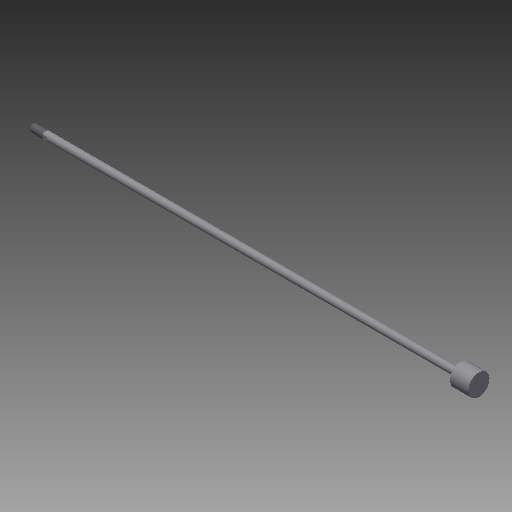
# Autodesk Inventor part: SR-1222-DP0000_rod
Saved by Autodesk Inventor 2019 (Build 230136000, 136)
## iProperties
Category: PARTsolutions
Company: BIMBA
Created: 2019-01-13
Part Number: SR-1222-DP0000_rod
Material: Generic
Catalog Web Link: www.cadenas.de
Description: Standard Air Cylinder_rod-Original Line - Standard Air Cylinders
Vendor: BIMBA
Document SubType Name: Modeling
Designer: psadmin
Manufacturer: BIMBA
Mass: 83.0612 g
Surface Area: 264.5 cm^2
Volume: 83.0612 cm^3
Density: 1 g/cm^3
Appearance: PSOLRGB-181-181-181
PSOL_IDENT_0: {$CADENAS_DATA\23d-libs\bimba\bimba\bimba_imperial\bimba_full_line\original_line_cylinders\standard_
PSOL_IDENT_1: air_cylinders\rod.prj},329 {VTYP=3D},{NB=SR-1222-DP0000_rod},{LINA=SR-1222-DP0000_rod},{NN=Standard
PSOL_IDENT_2: Air Cylinder_rod},{DATE=21.03.2018 14:31:21},{GEOMDATE=09.11.2017 13:09:15},{VERSION=},{LINEID=70},{
PSOL_IDENT_3: WBVAR=STROKE,ACTING,MNT,DER,NR,BM,CO,M,EE,EEL,K,Q,Y,F,G,T,B,H,SER,SR,NT,W,E,HL,ST,STP,PRC,PB,COLOR1,
PSOL_IDENT_4: FCD,RCD,BCD},{WBNUMERIC=STROKE,EEL,COLOR1,FCD,RCD,BCD}  {NB=SR-1222-DP0000_rod},{LINA=SR-1222-DP0000
PSOL_IDENT_5: _rod},{KT=DUMMY},{PN=SR-1222-DP000},{DASH=-},{BORE=1.25000000},{BOREPN=12},{STROKE=22.000},{STROKEAL
PSOL_IDENT_6: G=[0.001:50/0.001]},{STROKE1=22.000},{ACTING=D},{ACTINGALG= '' , 'Single Acting' , 'R' , 'Reverse Si
PSOL_IDENT_7: ngle Acting' , 'D' , 'Double Acting' },{ACTINGPN=D},{MNT=P},{MNTALG= '' , 'Front Nose Mounting' , 'P'
PSOL_IDENT_8: , 'Rear Pivot Mounting' , 'X' , 'Double End Mounting' },{TYPE=SR-},{MNTPN=P},{DER=},{DERALG= '' , '
PSOL_IDENT_9: N/A' },{NR=},{NRALG= '' , 'N/A' },{NRPN=},{BM=},{BMALG= '' , 'N/A' },{BMPN=},{CO=},{COALG= '' , 'N/A'
PSOL_IDENT_10: },{M=},{MALG= '', 'Without Magnet', 'M', 'With Magnet' },{EE=},{EEL=0},{EEMAX=28},{EEALG= '', 'With
PSOL_IDENT_11: out Extra Extension', 'EE', 'With Extra Extension' },{EELALG=0},{EEPN=},{EEPN1=0.000},{K=},{KALG= ''
PSOL_IDENT_12: , 'Standard' , 'K' , 'Ports Rotated 90deg' },{KPN=},{Q=},{QALG= '' , 'Without Side Ported Rear Head'
PSOL_IDENT_13: , 'Q' , 'With Side Ported Rear Head' },{QPN=},{Y=},{YALG= '' , 'Without Pivot Bushing' , 'Y' , 'Wit
PSOL_IDENT_14: h Pivot Bushing' },{YPN=},{F=},{FALG= '', 'Standard', 'F', 'Molycoated Body' },{FPN=},{G=},{GPN=},{T=
PSOL_IDENT_15: },{TALG= '' , 'Standard' , 'N' , 'Low Temperature' , 'V' , 'High Temperature' },{NPN=},{VPN=},{B=},{
PSOL_IDENT_16: BALG= '' , 'With Bumper' },{BPN=},{H=},{HALG= '', 'N/A' },{HPN=},{SER=},{SERALG= '' , 'Without Sprin
PSOL_IDENT_17: g Extend/Return' , 'JS' , 'With Spring Return' , 'JR' , 'With Spring Extend' },{SR=SR},{SRALG= 'C' ,
PSOL_IDENT_18: 'Carbon Steel Rod' , 'SR' , '303 Stainless Steel Rod' , '' , '303 Stainless Steel Rod1' },{SRPN=SR}
PSOL_IDENT_19: ,{SRCON=1},{NT=},{NTPN=},{W=},{WALG= '' , 'Without Wiper' , 'W' , 'With Wiper' },{WPN=},{E=},{EALG= ''
PSOL_IDENT_20: , 'Without Special Lube and Seals' , 'E' , 'With Special Lube and Seals' },{EPN=},{HL=},{HLALG= ''
PSOL_IDENT_21: , 'Wihout Low Pressure Hydraulic' , 'HL' , 'With Low Pressure Hydraulic' },{ST=},{STALG= '' , 'Witho
PSOL_IDENT_22: ut Switch Track' , 'T' , 'With Switch Track' },{STP=},{STPALG= '' , 'N/A' },{STPN=},{PRC=},{PRCALG= ''
PSOL_IDENT_23: , 'Without Piston Rod Clevis' , 'D-166-1' , 'With Piston Rod Clevis' },{PRCPN=},{PB=},{PBALG= '' , '
PSOL_IDENT_24: Without Pivot Bracket' , 'D-167' , 'With Pivot Bracket' },{PBPN=},{TLEN=23.4865},{TEXT=1.566667},{SP
PSOL_IDENT_25: ACE=0.895238},{FRAC=509.7200},{RGCON=},{RGDACCON=R},{RHCON=P},{RHCONON=1},{RHACCON=},{FNUTCON=1},{RN
PSOL_IDENT_26: UTCON=1},{FNUTPN=D-3556},{RNUTPN=D-3556},{FNUTTRANS=0.0000},{RNUTTRANS=0.0000},{VHOLECON=0},{A1=2.00
PSOL_IDENT_27: 00},{A1N=1.5620},{A1P=2.0000},{A1B=0.0000},{A4=0.2525},{A4N=0.6280},{A4P=0.2525},{A5=0.0400},{A1H=1.
PSOL_IDENT_28: 812},{A1NH=0.6880},{A1PH=1.8120},{A1BH=0.0000},{A1SH=1.1250},{A2H=0.2500},{A2NH=0.2500},{LENGTH=4.72
PSOL_IDENT_29: 00},{LENGTH1=4.7200},{LENGTH2=5.0900},{MUL=22.0000},{MUL11=22.0000},{MUL22=61.8200},{MUL33=39.8200},
PSOL_IDENT_30: {MUL2=22.0000},{MUL211=22.0000},{MUL222=2.8100},{MUL233=1.8100},{SSS=44.0000},{RGLEN=1.7875},{RHLEN=
PSOL_IDENT_31: 1.1960},{SSS1=23.0000},{A13=1.4060},{THDLEN1=0.7500},{THD1=0.4375},{TAB=UNF},{THDLEN=0.7500},{THD=0.
PSOL_IDENT_32: 4375},{OD=1.2615},{RODL=26.0640},{PL=1.0640},{RODDIA=0.4370},{HEX=0.4370},{RODTRANS=0.0000},{G1=0.37
PSOL_IDENT_33: 50},{ON=0},{G5=1.0000},{DERLEN=24.7500},{THOLE=0.2500},{WF=0.3800},{BADD=0.0000},{MADD=0.0000},{NVAD
PSOL_IDENT_34: D=0.000},{JRADD=0.00000},{COLOR=0.71,0.71,0.71,0.00},{GROOVE=1},{HOL=1},{D7=0.2525},{H1=1.3265},{D1=
PSOL_IDENT_35: 1.3265},{D1RH=1.3265},{D1P=0.0000},{D1B=1.3265},{D1N=1.3265},{D1NRH=1.3265},{D1BRH=0.0000},{D1PRH=1.
PSOL_IDENT_36: 3265},{BOZO=0},{HADD=0.000},{COLOR1=0},{DEFL=0.0000},{HEXL=0.0000},{SSADD=0.0000},{WFL=0.2500},{MOVE=
PSOL_IDENT_37: 0.2500},{PRCL2=0.75000},{PRCB=0.25000},{PRCTRANS=0.25000},{FCD=0},{RCD=0},{BCD=0}
NN: Standard Air Cylinder_rod
NT: Standard
NB: SR-1222-DP0000_rod
NBSYN: $PN.$COLOR1._rod
LINA: SR-1222-DP0000_rod
PN: SR-1222-DP000
BORE: 1.25
BOREPN: 12
STROKE: 22
ACTING: Double Acting
MNT: Rear Pivot Mounting
DER: N/A
NR: N/A
BM: N/A
CO: N/A
M: Without Magnet
EE: Without Extra Extension
EEL: 0
K: Standard
Q: Without Side Ported Rear Head
Y: Without Pivot Bushing
F: Standard
G: Without Magnalube Lubrication
T: Standard
B: With Bumper
H: N/A
SER: Without Spring Extend/Return
SR: 303 Stainless Steel Rod
W: Without Wiper
E: Without Special Lube and Seals
HL: Wihout Low Pressure Hydraulic
ST: Without Switch Track
STP: N/A
PRC: Without Piston Rod Clevis
PB: Without Pivot Bracket
A1N: 1.562
A1P: 2
A1B: 0
A4N: 0.628
A4P: 0.2525
A5: 0.04
A1NH: 0.688
A1PH: 1.812
A1BH: 0
A1SH: 1.125
A2NH: 0.25
A13: 1.406
THDLEN1: 0.75
THD1: 0.4375
TAB: UNF
OD: 1.2615
RODDIA: 0.437
HEX: 0.437
G1: 0.375
G5: 1
THOLE: 0.25
WF: 0.38
GROOVE: 1
D7: 0.2525
D1P: 0
D1B: 1.3265
D1N: 1.3265
D1NRH: 1.3265
D1BRH: 0
D1PRH: 1.3265
COLOR1: 0
FCD: 0
RCD: 0
BCD: 0
SUPPLIER: BIMBA
ARTICLENO: SR-1222-DP0000_rod
BOMINFO: SR-1222-DP0000_rod
CREATOR: CADENAS GmbH
Title: SR-1222-DP0000_rod
Author: Cadenas PARTsolutions
Comments: Original Line - Standard Air Cylinders
Autodesk Inventor part; units mm, degrees
sketch "Sketch_1" plane through (0, 0, 0) normal (0, 0, 1) x (1, 0, 0)
  line L0 (636.6256, 0) -> (-6.35, 0)
  line L1 (-6.35, 0) -> (-6.35, 5.5499)
  line L2 (-6.35, 5.5499) -> (609.6, 5.5499)
  line L3 (609.6, 5.5499) -> (609.6, 15.9703)
  line L4 (609.6, 15.9703) -> (636.6256, 15.9703)
  line L5 (636.6256, 15.9703) -> (636.6256, 0)
  line L6 (636.6256, 0) -> (-6.35, 0)
  constraints: 14 end point
revolve "Revolution1" add sketch "Sketch_1" angle 360 about axis through (636.6256, 0, 0) along (1, 0, 0)
sketch "Sketch_3" plane through (0, 0, 0) normal (0, 0, 1) x (1, 0, 0)
  line L0 (-6.35, 0) -> (-25.4, 0)
  line L1 (-25.4, 0) -> (-25.4, 4.8006)
  line L2 (-25.4, 4.8006) -> (-24.6443, 5.5563)
  line L3 (-24.6443, 5.5563) -> (-6.35, 5.5563)
  line L4 (-6.35, 5.5563) -> (-6.35, 0)
  line L5 (-6.35, 0) -> (-25.4, 0)
  constraints: 12 end point
revolve "Revolution2" add sketch "Sketch_3" angle 360 about axis through (-6.35, 0, 0) along (1, 0, 0)
thread "Thread1" size "7/16-20 UNF" class "2A" standard "ANSI Unified Screw Threads" full length
sketch "Sketch_10" plane through (-6.35, 0, 0) normal (1, 0, 0) x (0, 0, -1)
  line L0 (-11.0998, -11.0998) -> (11.0998, -11.0998)
  line L1 (11.0998, -11.0998) -> (11.0998, 11.0998)
  line L2 (11.0998, 11.0998) -> (-11.0998, 11.0998)
  line L3 (-11.0998, 11.0998) -> (-11.0998, -11.0998)
  line L4 (-4.826, -5.5499) -> (4.826, -5.5499)
  line L5 (4.826, -5.5499) -> (4.826, 5.5499)
  line L6 (4.826, 5.5499) -> (-4.826, 5.5499)
  line L7 (-4.826, 5.5499) -> (-4.826, -5.5499)
  constraints: 16 end point
extrude "Extrusion1" cut sketch "Sketch_10" along normal blind 6.35
ref_plane "dia1_XY" through (-6.35, 5.5499, 0) normal (1, 0, 0) x (0, 0, -1)
ref_plane "dia1_YZ" through (-6.35, 5.5499, 0) normal (0, 0, -1) x (0, 1, 0)
ref_plane "dia1_ZX" through (-6.35, 5.5499, 0) normal (0, 1, 0) x (1, 0, 0)
ref_plane "dia12_XY" through (0, 0, 16.8466) normal (1, 0, 0) x (0, 0, -1)
ref_plane "dia12_YZ" through (0, 0, 16.8466) normal (0, 0, -1) x (0, 1, 0)
ref_plane "dia12_ZX" through (0, 0, 16.8466) normal (0, 1, 0) x (1, 0, 0)
ref_plane "dia2_XY" through (-6.35, -5.5499, 0) normal (1, 0, 0) x (0, 0, -1)
ref_plane "dia2_YZ" through (-6.35, -5.5499, 0) normal (0, 0, -1) x (0, 1, 0)
ref_plane "dia2_ZX" through (-6.35, -5.5499, 0) normal (0, 1, 0) x (1, 0, 0)
ref_plane "dia22_XY" through (0, 0, -16.8466) normal (1, 0, 0) x (0, 0, -1)
ref_plane "dia22_YZ" through (0, 0, -16.8466) normal (0, 0, -1) x (0, 1, 0)
ref_plane "dia22_ZX" through (0, 0, -16.8466) normal (0, 1, 0) x (1, 0, 0)
ref_plane "hh1_XY" through (669.1313, 0, 0) normal (0, 0, 1) x (1, 0, 0)
ref_plane "hh1_YZ" through (669.1313, 0, 0) normal (1, 0, 0) x (0, 1, 0)
ref_plane "hh1_ZX" through (669.1313, 0, 0) normal (0, 1, 0) x (0, 0, 1)
ref_plane "hh2_XY" through (675.5448, 0, 0) normal (0, 0, 1) x (1, 0, 0)
ref_plane "hh2_YZ" through (675.5448, 0, 0) normal (1, 0, 0) x (0, 1, 0)
ref_plane "hh2_ZX" through (675.5448, 0, 0) normal (0, 1, 0) x (0, 0, 1)
ref_plane "rl1_XY" through (-25.4, 0, 0) normal (1, 0, 0) x (0, 0, -1)
ref_plane "rl1_YZ" through (-25.4, 0, 0) normal (0, 0, -1) x (0, 1, 0)
ref_plane "rl1_ZX" through (-25.4, 0, 0) normal (0, 1, 0) x (1, 0, 0)
ref_plane "rl2_XY" through (-6.35, 0, 0) normal (1, 0, 0) x (0, 0, -1)
ref_plane "rl2_YZ" through (-6.35, 0, 0) normal (0, 0, -1) x (0, 1, 0)
ref_plane "rl2_ZX" through (-6.35, 0, 0) normal (0, 1, 0) x (1, 0, 0)
ref_plane "rod_cp_XY" through (0, 0, 0) normal (1, 0, 0) x (0, 0, -1)
ref_plane "rod_cp_YZ" through (0, 0, 0) normal (0, 0, -1) x (0, 1, 0)
ref_plane "rod_cp_ZX" through (0, 0, 0) normal (0, 1, 0) x (1, 0, 0)
ref_plane "thd1_XY" through (-25.4, 5.5563, 0) normal (1, 0, 0) x (0, 0, -1)
ref_plane "thd1_YZ" through (-25.4, 5.5563, 0) normal (0, 0, -1) x (0, 1, 0)
ref_plane "thd1_ZX" through (-25.4, 5.5563, 0) normal (0, 1, 0) x (1, 0, 0)
ref_plane "thd2_XY" through (-25.4, -5.5563, 0) normal (1, 0, 0) x (0, 0, -1)
ref_plane "thd2_YZ" through (-25.4, -5.5563, 0) normal (0, 0, -1) x (0, 1, 0)
ref_plane "thd2_ZX" through (-25.4, -5.5563, 0) normal (0, 1, 0) x (1, 0, 0)
ref_plane "to_rod_clevis_XY" through (-31.75, 0, 0) normal (1, 0, 0) x (0, 0, -1)
ref_plane "to_rod_clevis_YZ" through (-31.75, 0, 0) normal (0, 0, -1) x (0, 1, 0)
ref_plane "to_rod_clevis_ZX" through (-31.75, 0, 0) normal (0, 1, 0) x (1, 0, 0)
ref_plane "wf1_XY" through (-6.35, 0, 0) normal (1, 0, 0) x (0, 0, -1)
ref_plane "wf1_YZ" through (-6.35, 0, 0) normal (0, 0, -1) x (0, 1, 0)
ref_plane "wf1_ZX" through (-6.35, 0, 0) normal (0, 1, 0) x (1, 0, 0)
ref_plane "wf2_XY" through (0, 0, 0) normal (1, 0, 0) x (0, 0, -1)
ref_plane "wf2_YZ" through (0, 0, 0) normal (0, 0, -1) x (0, 1, 0)
ref_plane "wf2_ZX" through (0, 0, 0) normal (0, 1, 0) x (1, 0, 0)
ref_plane "wfw1_XY" through (-6.35, 0, -4.826) normal (0, 1, 0) x (1, 0, 0)
ref_plane "wfw1_YZ" through (-6.35, 0, -4.826) normal (1, 0, 0) x (0, 0, -1)
ref_plane "wfw1_ZX" through (-6.35, 0, -4.826) normal (0, 0, -1) x (0, 1, 0)
ref_plane "wfw2_XY" through (-6.35, 0, 4.826) normal (0, 1, 0) x (1, 0, 0)
ref_plane "wfw2_YZ" through (-6.35, 0, 4.826) normal (1, 0, 0) x (0, 0, -1)
ref_plane "wfw2_ZX" through (-6.35, 0, 4.826) normal (0, 0, -1) x (0, 1, 0)
body "Solid1"
